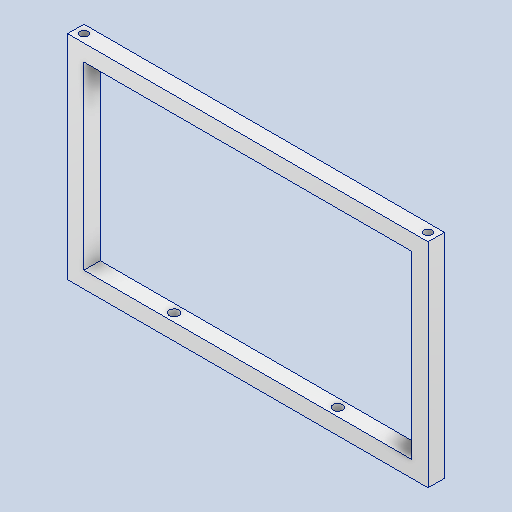
# Autodesk Inventor part: Camera plate shell
Saved by Autodesk Inventor 2023 (Build 270158000, 158)
## iProperties
Created: 2023-04-09
Part Number: Camera plate shell
Material: Aluminum 6061
Document SubType Name: Modeling
Designer: ASARe-DAQ-PC
Density: 2.7 g/cm^3
Appearance: Aluminum - Flat
Mass: 21.8983 g
Surface Area: 67.7571 cm^2
Volume: 8.11049 cm^3
Author: ASARe-DAQ-PC
Autodesk Inventor part; units mm, degrees
ref_plane "YZ Plane" through (0, 0, 0) normal (1, 0, 0) x (0, 1, 0)
ref_plane "XZ Plane" through (0, 0, 0) normal (0, 1, 0) x (-1, 0, 0)
ref_plane "XY Plane" through (0, 0, 0) normal (0, 0, 1) x (1, 0, 0)
sketch "Sketch1" plane through (0, 0, 0) normal (0, 0, 1) x (1, 0, 0)
  line L0 (0, 0) -> (110, 0)
  line L1 (110, 0) -> (110, 65)
  line L2 (110, 65) -> (0, 65)
  line L3 (0, 65) -> (0, 0)
  line L4 (5, 5) -> (105, 5)
  line L5 (105, 5) -> (105, 60)
  line L6 (105, 60) -> (5, 60)
  line L7 (5, 60) -> (5, 5)
  dimension "d0" = 65
  dimension "d1" = 110
  dimension "d4" = 5
  constraints: 16 end point, 4 parallel, 2 perpendicular, 1 horizontal, 3 other
  measures "d0" distance of L0.end L1.end
  measures "d1" distance of L1.end L2.end
  measures "d4" distance between parallel lines of L3 L7
extrude "Extrusion1" add sketch "Sketch1" along normal blind 5 contours L3 L2 L1 L0 | L7 L6 L5 L4
extrude "Extrusion2" cut sketch "Sketch1" along normal blind 5 contours L7 L6 L5 L4
sketch "Sketch2" plane through (0, 65, 0) normal (0, 1, 0) x (1, 0, 0)
  line L0 (110, 0) -> (110, -5) projected
  line L1 (110, 0) -> (0, 0) projected
  line L2 (0, 0) -> (0, -5) projected
  point P0 (2.5, -2.5)
  point P1 (107.5, -2.5)
  dimension "d14" = 2.5
  dimension "d15" = 2.5
  dimension "d16" = 2.5
  dimension "d17" = 2.5
  measures "d14" distance from line of L0 point (107.5, -2.5)
  measures "d15" distance from line of L1 point (107.5, -2.5)
  measures "d16" distance from line of L1 point (2.5, -2.5)
  measures "d17" distance from line of L2 point (2.5, -2.5)
hole "Hole1" at (2.5, 65, 2.5) at (107.5, 65, 2.5) direction (0, -1, 0) diameter 2.459 depth 7 tip angle 118 thread size "M3x0.5" class "6H" standard "ISO Metric profile"
sketch "Sketch4" plane through (5, 5, 0) normal (0, 1, 0) x (1, 0, 0)
  line L0 (0, 0) -> (0, -5) construction
  line L1 (0, -2.5) -> (100, -2.5) construction
  line L2 (100, 0) -> (100, -5) construction
  point P0 (-5, 0)
  point P1 (75, -2.5)
  point P2 (25, -2.5)
  dimension "d36" = 25
  dimension "d37" = 25
  constraints: 2 end point, 2 midpoint, 2 point on line
  measures "d36" distance from line of L0 point (25, -2.5)
  measures "d37" distance from line of L2 point (75, -2.5)
hole "Hole3" at (80, 5, 2.5) at (30, 5, 2.5) direction (0, -1, 0) diameter 3 depth 8.8 tip angle 118
body "Solid1"
